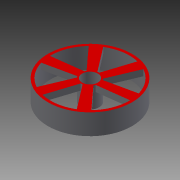
# Autodesk Inventor part: Part3
Saved by Autodesk Inventor 2015 (Build 190159000, 159)
## iProperties
Created: 2014-10-30
Part Number: Part3
Material: Generic
Document SubType Name: Modeling
Designer: hlorenson909
Density: 1 g/cm^3
Appearance: Default
Author: hlorenson909
Autodesk Inventor part; units mm, degrees
ref_plane "YZ Plane" through (0, 0, 0) normal (1, 0, 0) x (0, 1, 0)
ref_plane "XZ Plane" through (0, 0, 0) normal (0, 1, 0) x (-1, 0, 0)
sketch "Sketch1" plane through (0, 0, 0) normal (0, 0, 1) x (1, 0, 0)
  circle A0 centre (0, 0) radius 3.81
  circle A1 centre (0, 0) radius 4.4866
  circle A2 centre (0, 0) radius 20.32
  circle A3 centre (0, 0) radius 19.017
  dimension "d0" = 7.62
  dimension "d1" = 40.64
  constraints: 4 centre point, 2 coincident
  measures "d0" diameter of A0
  measures "d1" diameter of A2
extrude "Extrusion1" add sketch "Sketch1" against normal blind 10
ref_plane "Work Plane1" through (0, 0, 0) normal (0, 0, 1) x (1, 0, 0)
sketch "Sketch2" plane through (0, 0, 0) normal (0, 0, 1) x (1, 0, 0)
  circle A0 centre (0, 0) radius 4.4866 projected
  circle A1 centre (0, 0) radius 19.017 projected
  line L0 (0, 4.4866) -> (4.4866, 18.4802)
  line L1 (3.4, 2.9274) -> (9.1521, 16.6699)
  constraints: 4 end point, 4 point on circle
extrude "Extrusion2" add sketch "Sketch2" against normal blind 3 contours A0 L0 A1 L1 picked at (3.8455, 13.626)
pattern_circular "Circular Pattern1" count 6 over 360 about axis through (0, 0, 0) along (0, 0, -1) of "Extrusion2"
body "Solid1"
